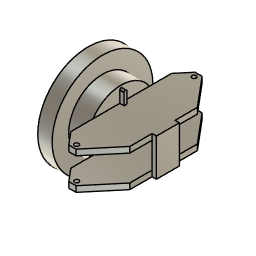
ITEM 3 v1 (Autodesk Fusion 360 design; units mm, degrees)
Autodesk Fusion 360 part; units mm, degrees
sketch "Sketch1" plane through (0, 0, 0) normal (1, 0, 0) x (0, 1, 0)
  circle A0 centre (0, 0) radius 35
  dimension "d1" = 70
  constraint coincident A0.centre origin
  measures "d1" diameter of A0
extrude "Extrude1" add sketch "Sketch1" along normal blind 10 in component "Component"
sketch "Sketch2" plane through (10, 0, 0) normal (1, 0, 0) x (0, 1, 0)
  circle A0 centre (0, 0) radius 35
  circle A1 centre (0, 0) radius 23.5
  dimension "d4" = 47
  constraint coincident A0.centre A1.centre
  measures "d4" diameter of A1
extrude "Extrude2" add sketch "Sketch2" along normal blind 13 contours A1 in component "Component"
ref_plane "WorkPlane1" through (0, 0, 13) normal (0, 0, 1) x (1, 0, 0)
sketch "Sketch3" plane through (0, 0, 13) normal (0, 0, 1) x (1, 0, 0)
  line L0 (23, 0) -> (23, -35)
  line L1 (23, -35) -> (23, -45)
  line L2 (23, -35) -> (30.3921, -43.8095)
  line L3 (23, -35) -> (34.5, -35) construction
  line L4 (23, 0) -> (60, 0)
  line L5 (23, -23.4992) -> (67, -23.4992)
  line L6 (30.3921, -43.8095) -> (35.3921, -43.8095)
  line L7 (35.3921, -43.8095) -> (52.4344, -23.4992)
  line L8 (35.3921, -43.8095) -> (45, -43.8095)
  line L9 (52.4344, -23.4992) -> (52.4344, 0)
  line L10 (23, 0) -> (23, 35)
  line L11 (23, 35) -> (30.3921, 43.8095)
  line L12 (30.3921, 43.8095) -> (35.3921, 43.8095)
  line L13 (52.4344, 23.4992) -> (52.4344, 0)
  line L14 (35.3921, 43.8095) -> (52.4344, 23.4992)
  dimension "d8" = 35
  dimension "d9" = 10
  dimension "d10" = 50
  dimension "d11" = 11.5
  dimension "d13" = 37
  dimension "d14" = 44
  dimension "d15" = 5
  dimension "d16" = 50
  constraint vertical L0
  constraint parallel L0 L1
  constraint horizontal L3
  constraint perpendicular L0 L4
  constraint coincident L0 L5.start
  constraint perpendicular L0 L5
  constraint horizontal L6
  constraint coincident L5 L7.end
  constraint parallel L5 L8
  constraint coincident L4 L9.end
  constraint perpendicular L4 L9
  constraint symmetric L0.start L4 L10.start
  constraint symmetric L0.end L4 L10.end
  constraint symmetric L2.end L4 L11.end
  constraint symmetric L4 L6.end L12.end
  constraint symmetric L4 L7.end L13.start
  constraint symmetric L4 L9.end L13.end
  measures "d8" distance of L0.start L0.end
  measures "d9" distance of L0.end L1.end
  measures "d10" angle of L2 L3
  measures "d11" distance of L0.end L2.end
  measures "d13" distance of L0.start L4.end
  measures "d14" distance of L5.start L5.end
  measures "d15" distance of L2.end L6.end
  measures "d16" angle of L7 L8
extrude "Extrude3" add sketch "Sketch3" against normal blind 4 in component "Component"
sketch "Sketch4" plane through (0, 0, 13) normal (0, 0, 1) x (-1, 0, 0)
  line L0 (-23, -35) -> (-23, -19.5768)
  line L1 (-23, -19.5768) -> (-23, 19.5768)
  line L2 (-23, 19.5768) -> (-23, 35)
  line L3 (-23, 35) -> (-30.3921, 43.8095)
  line L4 (-30.3921, 43.8095) -> (-35.3921, 43.8095)
  line L5 (-35.3921, 43.8095) -> (-52.4344, 23.4992)
  line L6 (-52.4344, 23.4992) -> (-52.4344, -23.4992)
  line L7 (-52.4344, -23.4992) -> (-35.3921, -43.8095)
  line L8 (-35.3921, -43.8095) -> (-30.3921, -43.8095)
  line L9 (-30.3921, -43.8095) -> (-23, -35)
  line L10 (-32.8921, 43.8095) -> (-32.8921, 40.8095)
  circle A0 centre (-32.8921, 40.8095) radius 1.5
  dimension "d19" = 3
  dimension "d20" = 3
  constraint midpoint L4 L10.start
  constraint perpendicular L4 L10
  constraint coincident L10.end A0.centre
  measures "d19" distance of L10.start L10.end
  measures "d20" diameter of A0
extrude "Extrude4" cut sketch "Sketch4" against normal blind 7 contours A0 in component "Component"
mirror "Mirror1" about plane through (0, 0, 0) normal (0, 1, 0) of "Extrude4" in component "Component"
mirror "Mirror2" about plane through (0, 0, 0) normal (0, 0, 1) of "Extrude3", "Extrude4", "Mirror1" in component "Component"
sketch "Sketch5" plane through (23, 0, 0) normal (1, 0, 0) x (0, 1, 0)
  line L0 (-19.5768, 13) -> (19.5768, 13)
  arc A0 (19.5768, 13) -> (-19.5768, 13) centre (0, 0) ccw
  line L1 (0, 13) -> (0, 23.5)
  line L2 (0, 13) -> (-1, 13)
  line L3 (-1, 13) -> (-1, 22)
  line L4 (-1, 22) -> (1, 22)
  line L5 (1, 22) -> (1, 13)
  constraint midpoint L0 L1.start
  constraint midpoint A0 L1.end
  constraint coincident L0 L2.end
  constraint perpendicular L2 L3
  constraint perpendicular L1 L4
  constraint coincident L0 L5.end
  constraint perpendicular L0 L5
extrude "Extrude5" add sketch "Sketch5" along normal blind 3 contours L0 L1 L2 L3 L4 | L0 L1 L4 L5 in component "Component"
fillet "Fillet1" radius 1 2 edges at (24.5, 1, 22) (24.5, -1, 22) in component "Component"
mirror "Mirror3" about plane through (0, 0, 0) normal (0, 0, 1) of "Extrude5", "Fillet1" in component "Component"
sketch "Sketch6" plane through (52.4344, 0, 0) normal (1, 0, 0) x (0, 1, 0)
  line L0 (23.4992, 13) -> (-23.4992, 13)
  line L1 (-23.4992, 13) -> (-23.4992, 9)
  line L2 (-23.4992, 9) -> (23.4992, 9)
  line L3 (23.4992, 9) -> (23.4992, 13)
  line L4 (8, -13) -> (-8, -13)
  line L5 (-8, -13) -> (-8, 13)
  line L6 (-8, 13) -> (8, 13)
  line L7 (8, 13) -> (8, -13)
  line L8 (8, -13) -> (-8, 13) construction
  line L9 (-8, -13) -> (8, 13) construction
  constraint horizontal L4
  constraint perpendicular L4 L5
  constraint parallel L4 L6
  constraint parallel L5 L7
  constraint coincident L8 origin
  constraint coincident L9 origin
extrude "Extrude6" add sketch "Sketch6" along normal blind 3 contours L0 L2 L5 L6 L7 | L2 L4 L5 L7 in component "Component"
sketch "Sketch7" plane through (0, 0, 0) normal (-1, 0, 0) x (0, -1, 0)
  circle A0 centre (0, 0) radius 35
  circle A1 centre (0, 0) radius 10
  dimension "d35" = 20
  constraint coincident A0.centre A1.centre
  measures "d35" diameter of A1
extrude "Extrude7" cut sketch "Sketch7" against normal blind 10 contours A1 in component "Component"
component "Component" placed x (1, 0, 0) y (0, 1, 0) z (0, 0, 1) at (0, 0, 0)
